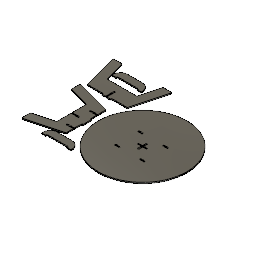
v2 (Autodesk Fusion 360 design; units mm, degrees)
Autodesk Fusion 360 part; units mm, degrees
sketch "Sketch1" plane through (0, 0, 0) normal (0, 1, 0) x (1, 0, 0) in component "Fótur1"
  line L0 (100, -38.0981) -> (100, 161.9019) construction
  line L1 (0, 0) -> (67.8461, 0)
  line L2 (67.8461, 0) -> (100, 120)
  line L3 (-120, 120) -> (172.4, 120) construction
  line L4 (50.1853, 50) -> (68.9417, 120)
  line L5 (0, 50) -> (50.1853, 50)
  line L6 (0, -1.75) -> (0, -22.5)
  line L7 (68.9417, 120) -> (100, 120)
  line L8 (0, 0) -> (-67.8461, 0)
  line L9 (0, 50) -> (-50.1853, 50)
  line L10 (-50.1853, 50) -> (-68.9417, 120)
  line L11 (-67.8461, 0) -> (-100, 120)
  line L12 (-68.9417, 120) -> (-100, 120)
  dimension "d8" = 100
  dimension "d10" = 15
  dimension "d11" = 50
  dimension "d13" = 30
  dimension "d125" = 120
  constraint vertical L0
  constraint coincident L1.start L8.start
  constraint coincident L0 L2.end
  constraint horizontal L3
  constraint coincident L2.end L3
  constraint coincident L3 L4.end
  constraint parallel L2 L4
  constraint perpendicular L5 L6
  constraint coincident L5.start L6
  constraint symmetric L1.start L6 L8.start
  constraint symmetric L1.end L6 L8.end
  constraint symmetric L2.end L6 L11.end
  constraint symmetric L4.start L6 L9.end
  constraint symmetric L4.end L6 L10.end
  constraint symmetric L5.start L6 L9.start
  measures "d8" distance of L1.start L0
  measures "d10" angle of L0 L2
  measures "d11" distance of L1 L5
  measures "d13" distance of L2 L4
  measures "d125" distance of L3 L8
extrude "Extrude1" add sketch "Sketch1" along normal blind 4 makes body 1 in component "Fótur1"
fillet "Fillet1" radius 2.5 8 edges at (100, 2, -120) (68.9417, 2, -120) (67.8461, 2, 0) (50.1853, 2, -50) (-50.1853, 2, -50) (-68.9417, 2, -120) (-100, 2, -120) (-67.8461, 2, 0) on bodies 1 in component "Fótur1"
sketch "Sketch2" plane through (0, 0, 0) normal (0, 1, 0) x (1, 0, 0) in component "Fótur1"
  line L0 (-15, -4) -> (15, -4)
  line L1 (15, -4) -> (15, 0)
  line L2 (15, 0) -> (-15, 0)
  line L3 (-15, 0) -> (-15, -4)
  line L4 (0, -1.75) -> (0, -22.5)
  line L5 (65.9278, 0) -> (-65.9278, 0)
  dimension "d19" = 4
  dimension "d20" = 30
  constraint horizontal L0
  constraint vertical L1
  constraint horizontal L2
  constraint vertical L3
  constraint symmetric L1 L3 L4
  constraint collinear L2 L5
  measures "d19" distance of L0 L2
  measures "d20" distance of L0.start L0.end
extrude "Extrude2" add sketch "Sketch2" along normal up to surface (4 mm away) bodies 1 in component "Fótur1"
sketch "Sketch3" plane through (0, 0, 0) normal (0, -1, 0) x (1, 0, 0) in component "Fótur1"
  arc A0 (-65.9278, 0) -> (-68.3426, -1.853) centre (-65.9278, -2.5) ccw
  line L0 (-68.3426, -1.853) -> (-99.1568, -116.853)
  arc A1 (-99.1568, -116.853) -> (-96.7419, -120) centre (-96.7419, -117.5) ccw
  line L1 (-96.7419, -120) -> (-70.86, -120)
  arc A2 (-70.86, -120) -> (-68.4452, -118.147) centre (-70.86, -117.5) ccw
  line L2 (-68.4452, -118.147) -> (-50.6818, -51.853)
  arc A3 (-48.267, -50) -> (-50.6818, -51.853) centre (-48.267, -52.5) ccw
  line L3 (-48.267, -50) -> (48.267, -50)
  arc A4 (50.6818, -51.853) -> (48.267, -50) centre (48.267, -52.5) ccw
  line L4 (50.6818, -51.853) -> (68.4452, -118.147)
  arc A5 (68.4452, -118.147) -> (70.86, -120) centre (70.86, -117.5) ccw
  line L5 (70.86, -120) -> (96.7419, -120)
  arc A6 (96.7419, -120) -> (99.1568, -116.853) centre (96.7419, -117.5) ccw
  line L6 (99.1568, -116.853) -> (68.3426, -1.853)
  arc A7 (68.3426, -1.853) -> (65.9278, 0) centre (65.9278, -2.5) ccw
  line L7 (65.9278, 0) -> (15, 0)
  line L8 (15, 0) -> (15, 4)
  line L9 (15, 4) -> (-15, 4)
  line L10 (-15, 4) -> (-15, 0)
  line L11 (-15, 0) -> (-65.9278, 0)
  line L12 (-1.78, 4) -> (1.78, 4)
  line L13 (1.78, 4) -> (1.78, -24.78)
  line L14 (1.78, -24.78) -> (-1.78, -24.78)
  line L15 (-1.78, -24.78) -> (-1.78, 4)
  line L16 (0, 1.75) -> (0, 22.5)
  line L17 (-1.78, -24.78) -> (0.7408, -22.2592) construction
  circle A8 centre (-1.7022, -24.7022) radius 0.11
  circle A9 centre (1.7022, -24.7022) radius 0.11
  dimension "d24" = 28.78
  dimension "d27" = 3.56
  dimension "d34" = 45
  dimension "d35" = 0.22
  dimension "d36" = 0.11
  constraint horizontal L12
  constraint vertical L13
  constraint horizontal L14
  constraint vertical L15
  constraint coincident L9 L12.start
  constraint symmetric L13 L15 L16
  constraint coincident L17 A8.centre
  constraint symmetric L16 A8 A9
  measures "d24" distance of L12.start L14.end
  measures "d27" distance of L13.end L14.end
  measures "d34" angle of L14 L17
  measures "d35" diameter of A8
  measures "d36" distance of L14.end A8.centre
sketch "Sketch1 (2)" plane through (0, 0, 0) normal (0, 1, 0) x (1, 0, 0) in component "Fótur1 (1)"
  line L0 (100, -38.0981) -> (100, 161.9019) construction
  line L1 (0, 0) -> (67.8461, 0)
  line L2 (67.8461, 0) -> (100, 120)
  line L3 (-120, 120) -> (172.4, 120) construction
  line L4 (50.1853, 50) -> (68.9417, 120)
  line L5 (0, 50) -> (50.1853, 50)
  line L6 (0, -1.75) -> (0, -22.5)
  line L7 (68.9417, 120) -> (100, 120)
  line L8 (0, 0) -> (-67.8461, 0)
  line L9 (0, 50) -> (-50.1853, 50)
  line L10 (-50.1853, 50) -> (-68.9417, 120)
  line L11 (-67.8461, 0) -> (-100, 120)
  line L12 (-68.9417, 120) -> (-100, 120)
  dimension "d8_1" = 100
  dimension "d10_1" = 15
  dimension "d11_1" = 50
  dimension "d13_1" = 30
  dimension "d126" = 120
  constraint vertical L0
  constraint coincident L1.start L8.start
  constraint coincident L0 L2.end
  constraint horizontal L3
  constraint coincident L2.end L3
  constraint coincident L3 L4.end
  constraint parallel L2 L4
  constraint perpendicular L5 L6
  constraint coincident L5.start L6
  constraint symmetric L1.start L6 L8.start
  constraint symmetric L1.end L6 L8.end
  constraint symmetric L2.end L6 L11.end
  constraint symmetric L4.start L6 L9.end
  constraint symmetric L4.end L6 L10.end
  constraint symmetric L5.start L6 L9.start
  measures "d8_1" distance of L1.start L0
  measures "d10_1" angle of L0 L2
  measures "d11_1" distance of L1 L5
  measures "d13_1" distance of L2 L4
  measures "d126" distance of L3 L8
extrude "Extrude1'" add sketch "Sketch1 (2)" along normal mid plane 4 separate body makes body 2 in component "Fótur1 (1)"
fillet "Fillet1'" radius 2.5 8 edges at (100, 0, -120) (68.9417, 0, -120) (67.8461, 0, 0) (50.1853, 0, -50) (-50.1853, 0, -50) (-68.9417, 0, -120) (-100, 0, -120) (-67.8461, 0, 0) on bodies 2 in component "Fótur1 (1)"
sketch "Sketch2 (2)" plane through (0, 0, 0) normal (0, 1, 0) x (1, 0, 0) in component "Fótur1 (1)"
  line L0 (-15, -4) -> (15, -4)
  line L1 (15, -4) -> (15, 0)
  line L2 (15, 0) -> (-15, 0)
  line L3 (-15, 0) -> (-15, -4)
  line L4 (0, -1.75) -> (0, -22.5)
  line L5 (65.9278, 0) -> (-65.9278, 0)
  dimension "d19_1" = 4
  dimension "d20_1" = 30
  constraint horizontal L0
  constraint vertical L1
  constraint horizontal L2
  constraint vertical L3
  constraint symmetric L1 L3 L4
  constraint collinear L2 L5
  measures "d19_1" distance of L0 L2
  measures "d20_1" distance of L0.start L0.end
extrude "Extrude2'" add sketch "Sketch2 (2)" along normal mid plane 4 bodies 2 in component "Fótur1 (1)"
sketch "Sketch5" plane through (0, -2, 0) normal (0, -1, 0) x (1, 0, 0) in component "Fótur1 (1)"
  arc A0 (-65.9278, 0) -> (-68.3426, -1.853) centre (-65.9278, -2.5) ccw
  line L0 (-68.3426, -1.853) -> (-99.1568, -116.853)
  arc A1 (-99.1568, -116.853) -> (-96.7419, -120) centre (-96.7419, -117.5) ccw
  line L1 (-96.7419, -120) -> (-70.86, -120)
  arc A2 (-70.86, -120) -> (-68.4452, -118.147) centre (-70.86, -117.5) ccw
  line L2 (-68.4452, -118.147) -> (-50.6818, -51.853)
  arc A3 (-48.267, -50) -> (-50.6818, -51.853) centre (-48.267, -52.5) ccw
  line L3 (-48.267, -50) -> (48.267, -50)
  arc A4 (50.6818, -51.853) -> (48.267, -50) centre (48.267, -52.5) ccw
  line L4 (50.6818, -51.853) -> (68.4452, -118.147)
  arc A5 (68.4452, -118.147) -> (70.86, -120) centre (70.86, -117.5) ccw
  line L5 (70.86, -120) -> (96.7419, -120)
  arc A6 (96.7419, -120) -> (99.1568, -116.853) centre (96.7419, -117.5) ccw
  line L6 (99.1568, -116.853) -> (68.3426, -1.853)
  arc A7 (68.3426, -1.853) -> (65.9278, 0) centre (65.9278, -2.5) ccw
  line L7 (65.9278, 0) -> (15, 0)
  line L8 (-1.78, -25.22) -> (1.78, -25.22)
  line L9 (1.78, -25.22) -> (1.78, -50)
  line L10 (1.78, -50) -> (-1.78, -50)
  line L11 (-1.78, -50) -> (-1.78, -25.22)
  line L12 (-2, 1.75) -> (-2, 22.5)
  line L13 (0, 1.75) -> (0, 22.5)
  line L14 (-1.78, -25.22) -> (-0.3547, -26.6453) construction
  circle A8 centre (-1.7022, -25.2978) radius 0.11
  line L15 (1.78, -25.22) -> (0.3547, -26.6453) construction
  circle A9 centre (1.7022, -25.2978) radius 0.11
  line L16 (15, 0) -> (15, 4)
  line L17 (15, 4) -> (-15, 4)
  line L18 (-15, 4) -> (-15, 0)
  line L19 (-15, 0) -> (-65.9278, 0)
  dimension "d37" = 3.56
  dimension "d38" = 24.78
  dimension "d39" = 45
  dimension "d40" = 0.22
  dimension "d41" = 0.11
  constraint horizontal L8
  constraint vertical L9
  constraint horizontal L10
  constraint vertical L11
  constraint coincident L3 L9.end
  constraint coincident L14 A8.centre
  constraint symmetric L8.start L13 L8.end
  constraint symmetric L13 L14.end L15.end
  constraint symmetric L13 A8 A9
  measures "d37" distance of L9.end L10.end
  measures "d38" distance of L8.start L10.end
  measures "d39" angle of L8 L14
  measures "d40" diameter of A8
  measures "d41" distance of L8.start A8.centre
extrude "Extrude4" cut sketch "Sketch5" against normal blind 4 contours L3 L8 L9 L10 L11 A8 A9 | L11 A8 | L8 L11 A8 | L8 L9 A9 | L9 A9 | L8 A8 | L8 A9 bodies 2 in component "Fótur1 (1)"
sketch "Sketch6" plane through (0, 0, 0) normal (0, 1, 0) x (1, 0, 0) in component "Fótur1 (1)"
  line L0 (-15, -4) -> (15, -4)
  line L1 (37.5, -17.5842) -> (37.5, 15.9433) construction
  line L2 (35.72, 0) -> (39.28, 0)
  line L3 (39.28, 0) -> (39.28, 24.78)
  line L4 (39.28, 24.78) -> (35.72, 24.78)
  line L5 (35.72, 24.78) -> (35.72, 0)
  line L6 (35.72, 24.78) -> (50.0286, 10.4714) construction
  circle A0 centre (35.7978, 24.7022) radius 0.11
  circle A1 centre (39.2022, 24.7022) radius 0.11
  line L7 (65.9278, 0) -> (15, 0)
  dimension "d45" = 3.56
  dimension "d46" = 24.78
  dimension "d47" = 45
  dimension "d48" = 0.22
  dimension "d49" = 0.11
  dimension "d86" = 37.5
  constraint vertical L1
  constraint horizontal L2
  constraint vertical L3
  constraint horizontal L4
  constraint vertical L5
  constraint symmetric L1 L3 L5
  constraint coincident L6 A0.centre
  constraint symmetric L1 A0 A1
  constraint collinear L2 L7
  measures "d45" distance of L2.start L2.end
  measures "d46" distance of L2.start L4.end
  measures "d47" angle of L4 L6
  measures "d48" diameter of A0
  measures "d49" distance of L4.end A0.centre
  measures "d86" distance of origin L1
extrude "Extrude5" cut sketch "Sketch6" along normal up to surface (2 mm away) bodies 2 in component "Fótur1 (1)"
extrude "Extrude7" cut 1 faces at (36.9067, 0, -8.2081) along direction (0, -1, 0) blind 2 on bodies 2 bodies 2 in component "Fótur1 (1)"
mirror "Mirror2" about plane through (-2, 2, 0) normal (1, 0, 0) of "Extrude7" in component "Fótur1 (1)"
extrude "Extrude8" cut 1 faces at (-40.9067, 0, -8.2081) along direction (0, 1, 0) blind 2 on bodies 2 bodies 2 in component "Fótur1 (1)"
ref_plane "WorkPlane1" through (0, 0, 0) normal (0, 1, 0) x (0, 0, 1) in component "Stallur"
ref_plane "WorkPlane2" through (1, 39.5, -12.3122) normal (0, -1, 0) x (0, 0, 1) in component "Stallur"
sketch "Sketch1 (3)" plane through (0, 39.5, -12.3165) normal (0, -1, 0) x (1, 0, 0) in component "Stallur"
  line L0 (0, 12.3165) -> (-50, 12.3165)
  line L1 (-50, 12.3165) -> (-50, -12.6835)
  line L2 (-35, 16.3165) -> (-50, 16.3165)
  line L3 (-50, 16.3165) -> (-50, 12.3165)
  line L4 (-50, 12.3165) -> (-35, 12.3165)
  line L5 (-35, 12.3165) -> (-35, 16.3165)
  line L6 (0.0028, -12.6835) -> (-50, -12.6835)
  line L7 (0, 14.0665) -> (0, 34.8165)
  line L8 (-0.0028, -12.6835) -> (50, -12.6835)
  line L9 (50, 12.3165) -> (50, -12.6835)
  line L10 (35, 16.3165) -> (50, 16.3165)
  line L11 (50, 16.3165) -> (50, 12.3165)
  line L12 (35, 12.3165) -> (35, 16.3165)
  line L13 (0, 12.3165) -> (50, 12.3165)
  line L14 (-35, 12.3165) -> (-30.5053, 16.8112) construction
  circle A0 centre (-34.9222, 12.3943) radius 0.11
  circle A1 centre (34.9222, 12.3943) radius 0.11
  line L15 (50, 16.3165) -> (50, 12.3165)
  line L16 (35, 16.3165) -> (35, 12.3165)
  line L17 (-35, 16.3165) -> (-34.9222, 12.3943)
  line L18 (-50, 16.3165) -> (-50, 12.3165)
  point P0 (0, 12.3165)
  dimension "d68" = 15
  dimension "d69" = 4
  dimension "d70" = 50
  dimension "d71" = 25
  dimension "d75" = 45
  dimension "d76" = 0.22
  dimension "d77" = 0.11
  constraint horizontal L0
  constraint vertical L1
  constraint horizontal L2
  constraint vertical L3
  constraint horizontal L4
  constraint vertical L5
  constraint coincident P0 L0.start
  constraint perpendicular L1 L6
  constraint symmetric P0 L7 L0.start
  constraint symmetric L0.end L7 L9.start
  constraint symmetric L1.end L7 L8.end
  constraint symmetric L2.start L7 L10.start
  constraint symmetric L2.end L7 L10.end
  constraint symmetric L4.end L7 L12.start
  constraint symmetric L6.start L7 L8.start
  constraint coincident L14 A0.centre
  constraint symmetric L7 A0 A1
  constraint coincident A0.centre L17.end
  measures "d68" distance of L2.start L2.end
  measures "d69" distance of L0.end L2.end
  measures "d70" distance of origin L1
  measures "d71" distance of L0.end L1.end
  measures "d75" angle of L0 L14
  measures "d76" diameter of A0
  measures "d77" distance of L4.end A0.centre
extrude "Extrude1''" add sketch "Sketch1 (3)" along normal mid plane 4 separate body contours L0 L1 L4 L6 L8 L9 L13 A0 A1 | L0 L2 L3 L4 L5 A0 L18 | L10 L11 L12 L13 A1 L15 L16 makes body 3 in component "Stallur"
fillet "Fillet1''" radius 25 2 edges at (-50, 39.5, -25) (50, 39.5, -25) on bodies 3 in component "Stallur"
mirror "Mirror1" about plane through (0, 0, 0) normal (0, 1, 0) of bodies 3 makes body 4 in component "Stallur"
sketch "Sketch1 (4)" plane through (0, 0, 0) normal (0, 0, 1) x (1, 0, 0) in component "Diskur"
  circle A0 centre (2, 2) radius 150
  line L0 (0, -13) -> (0, 17)
  line L1 (16.785, 4) -> (-13.215, 4) construction
  line L2 (-13.215, 0) -> (16.785, 0) construction
  line L3 (4, 17) -> (4, -13)
  line L4 (4, 17) -> (0, 17) construction
  line L5 (0, 17) -> (0, -13) construction
  line L6 (0, -13) -> (4, -13)
  line L7 (4, -13) -> (4, 17) construction
  line L8 (4, -13) -> (0, -13) construction
  line L9 (-13.215, 4) -> (-13.215, 0) construction
  line L10 (16.785, 4) -> (16.785, 0) construction
  line L11 (16.565, 3.78) -> (16.565, 0.22)
  line L12 (-12.995, 0.22) -> (16.565, 0.22)
  line L13 (-12.995, 3.78) -> (-12.995, 0.22)
  line L14 (16.565, 3.78) -> (-12.995, 3.78)
  line L15 (3.78, -12.78) -> (3.78, 16.78)
  line L16 (3.78, 16.78) -> (0.22, 16.78)
  line L17 (0.22, 16.78) -> (0.22, -12.78)
  line L18 (0.22, -12.78) -> (3.78, -12.78)
  line L19 (-50, 41.5) -> (-50, 37.5) construction
  line L20 (-50, 37.5) -> (-35, 37.5) construction
  line L21 (-35, 37.5) -> (-35, 41.5) construction
  line L22 (-35, 41.5) -> (-50, 41.5) construction
  line L23 (-49.78, 37.72) -> (-35.22, 37.72)
  line L24 (-35.22, 37.72) -> (-35.22, 41.28)
  line L25 (-35.22, 41.28) -> (-49.78, 41.28)
  line L26 (-49.78, 41.28) -> (-49.78, 37.72)
  line L27 (0, 1.75) -> (0, 22.5)
  line L28 (35.22, 41.28) -> (49.78, 41.28)
  line L29 (35.22, 37.72) -> (35.22, 41.28)
  line L30 (49.78, 37.72) -> (35.22, 37.72)
  line L31 (49.78, 41.28) -> (49.78, 37.72)
  line L32 (1.75, 0) -> (22.5, 0)
  line L33 (49.78, -37.72) -> (35.22, -37.72)
  line L34 (35.22, -37.72) -> (35.22, -41.28)
  line L35 (35.22, -41.28) -> (49.78, -41.28)
  line L36 (49.78, -41.28) -> (49.78, -37.72)
  line L37 (-49.78, -37.72) -> (-35.22, -37.72)
  line L38 (-35.22, -41.28) -> (-49.78, -41.28)
  line L39 (-35.22, -37.72) -> (-35.22, -41.28)
  line L40 (-49.78, -41.28) -> (-49.78, -37.72)
  dimension "d119" = 300
  dimension "d120" = 0.22
  constraint coincident L1.end L9.start
  constraint coincident L2.start L9.end
  constraint coincident L1.start L10.start
  constraint coincident L2.end L10.end
  constraint symmetric L23.start L27 L30.start
  constraint symmetric L23.end L27 L29.start
  constraint symmetric L24.end L27 L28.start
  constraint symmetric L25.end L27 L28.end
  constraint symmetric L23.start L32 L37.start
  constraint symmetric L23.end L32 L37.end
  constraint symmetric L24.end L32 L38.start
  constraint symmetric L25.end L32 L38.end
  constraint symmetric L28.start L32 L34.end
  constraint symmetric L28.end L32 L35.end
  constraint symmetric L29.start L32 L33.end
  constraint symmetric L30.start L32 L33.start
  measures "d119" diameter of A0
extrude "Extrude1'''" add sketch "Sketch1 (4)" along normal blind 4 separate body makes body 5 in component "Diskur"
extrude "Extrude5'" cut sketch "Sketch3" against normal blind 4 contours L9 L12 L13 L14 L15 A8 A9 | L14 L15 A8 | L15 A8 | L14 A8 | L13 A9 | L13 L14 A9 | L14 A9 bodies 1 in component "Fótur1"
fillet "Fillet2" radius 0.5 4 edges at (-39.72, 0, 0) (-43.28, 0, 0) (35.72, 0, 0) (39.28, 0, 0) on bodies 2 in component "Fótur1 (1)"
fillet "Fillet2'" radius 0.5 2 edges at (-1.78, 2, 4) (1.78, 2, 4) on bodies 1 in component "Fótur1"
fillet "Fillet3" radius 0.5 2 edges at (-1.78, 0, -50) (1.78, 0, -50) on bodies 2 in component "Fótur1 (1)"
move_body "Move1" bodies 4 to x (0, 0, -1) y (0, -1, 0) z (-1, 0, 0) at (-25, -75, -25) in component "Stallur"
move_body "Move2" bodies 4 to x (0, 0, -1) y (0, 1, 0) z (1, 0, 0) at (25, 0, -75) in component "Stallur"
component "3D-módel" placed x (1, 0, 0) y (0, 1, 0) z (0, 0, 1) at (0, 0, 0)
component "Smíðateikning" placed x (1, 0, 0) y (0, 1, 0) z (0, 0, 1) at (0, 0, 0)
component "Diskur" placed x (1, 0, 0) y (0, 1, 0) z (0, 0, 1) at (0, 0, 0) in component "3D-módel"
component "Fótur1" placed x (1, 0, 0) y (0, 1, 0) z (0, 0, 1) at (1.785, 0, 0) in component "3D-módel"
component "Fótur1 (1)" placed x (0, 1, 0) y (-1, 0, 0) z (0, 0, 1) at (2, 2, 0) in component "3D-módel"
component "Stallur" placed x (1, 0, 0) y (0, 1, 0) z (0, 0, 1) at (0, 0, 0) in component "3D-módel"
component "Diskur" placed x (1, 0, 0) y (0, 1, 0) z (0, 0, 1) at (0, 0, 0) in component "Smíðateikning"
component "Fótur1 (1)" placed x (0, 1, 0) y (0, 0, 1) z (1, 0, 0) at (2, 2, 2) in component "Smíðateikning"
component "Fótur1" placed x (1, 0, 0) y (0, 0, 1) z (0, -1, 0) at (1.785, 0, 0) in component "Smíðateikning"
component "Stallur" placed x (1, 0, 0) y (0, 0, 1) z (0, -1, 0) at (0, 0, 41.5) in component "Smíðateikning"
component "Stallur" placed x (1, 0, 0) y (0, 0, 1) z (0, -1, 0) at (0, 0, 41.5) in component "Smíðateikning"
hidden bodies 3
equation "Þvermál = 300 mm"
equation "Þykkt = 4 mm"
equation "Hæð = 120 mm"
equation "Dýpt_fótar = 50 mm"
equation "d8 = Þvermál / 3"
equation "d11 = Dýpt_fótar"
equation "Þykkt_fóta = 30 mm"
equation "d13 = Þykkt_fóta"
equation "d14 = Þykkt"
equation "Kantar = 2.5 mm"
equation "d18 = Kantar"
equation "d19 = Þykkt"
equation "d20 = Flipar_lengd"
equation "Flipar_lengd = 30 mm"
equation "d24 = Dýpt_fótar / 2 + Þykkt - Kerf"
equation "Slit = Þykkt - Kerf * 2"
equation "Kerf = 0.22 mm"
equation "d27 = Slit"
equation "d35 = Kerf"
equation "d36 = Kerf / 2"
equation "d8_1 = Þvermál / 3"
equation "d11_1 = Dýpt_fótar"
equation "d13_1 = Þykkt_fóta"
equation "d14_1 = Þykkt / 2"
equation "d18_1 = Kantar"
equation "d19_1 = Þykkt"
equation "d20_1 = Flipar_lengd"
equation "d37 = Slit"
equation "d38 = Dýpt_fótar / 2 - Kerf"
equation "d40 = Kerf"
equation "d41 = Kerf / 2"
equation "d45 = Slit"
equation "d46 = Dýpt_fótar / 2 - Kerf"
equation "d48 = Kerf"
equation "d49 = Kerf / 2"
equation "d68 = Flipar_lengd / 2"
equation "d69 = Þykkt"
equation "d70 = Þvermál / 6"
equation "d71 = Dýpt_fótar / 2"
equation "d72 = Þykkt / 2"
equation "Curve_stallur = 25 mm"
equation "d76 = Kerf"
equation "d77 = Kerf / 2"
equation "d79 = Curve_stallur"
equation "Endar = 0 mm"
equation "d86 = Þvermál / 8"
equation "d119 = Þvermál"
equation "d120 = Kerf"
equation "d121 = -Kerf"
equation "d122 = -Kerf"
equation "d123 = Þykkt"
equation "d125 = Hæð"
equation "d126 = Hæð"
equation "Endar_final = 0.5 mm"
equation "d131 = Endar_final"
equation "d133 = Endar_final"
equation "d135 = Endar_final"
